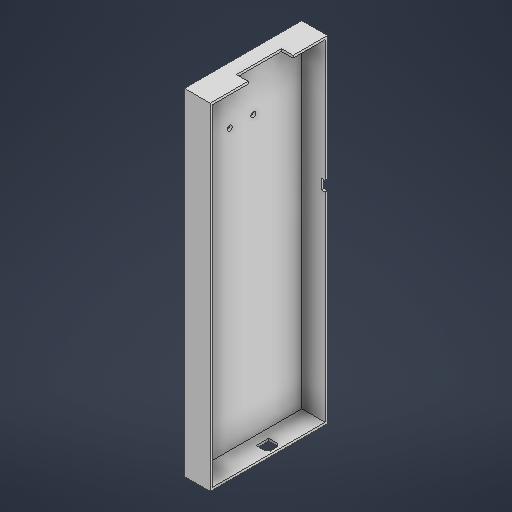
# Autodesk Inventor part: cDAQ_Bottom_Box3
Saved by Autodesk Inventor 2027 (Build 310192000, 192)
## iProperties
Created: 2026-05-08
Part Number: cDAQ_Bottom_Box3
Material: Generic
Document SubType Name: Modeling
Designer: giese
Density: 1 g/cm^3
Appearance: Default
Author: giese
Autodesk Inventor part; units mm, degrees
ref_plane "YZ Plane" through (0, 0, 0) normal (1, 0, 0) x (0, 1, 0)
ref_plane "XZ Plane" through (0, 0, 0) normal (0, 1, 0) x (-1, 0, 0)
ref_plane "XY Plane" through (0, 0, 0) normal (0, 0, 1) x (1, 0, 0)
sketch "Sketch1" plane through (0, 0, 0) normal (1, 0, 0) x (0, 1, 0)
  line L0 (37.5698, 44.2767) -> (-228.1396, 44.2767)
  line L1 (-228.1396, 44.2767) -> (-228.1396, -48.4333)
  line L2 (-228.1396, -48.4333) -> (37.5698, -48.4333)
  line L3 (37.5698, -48.4333) -> (37.5698, 44.2767)
  point P0 (0, 0)
  dimension "d0" = 92.71
  dimension "d1" = 265.7094
  constraints: 8 end point, 2 parallel, 1 horizontal, 1 perpendicular
  measures "d0" distance of L2.end L0.start
  measures "d1" distance of L1.end L2.end
extrude "Extrusion1" add sketch "Sketch1" along normal blind 20.32
sketch "Sketch2" plane through (20.32, 0, 0) normal (1, 0, 0) x (0, 0, -1)
  line L0 (46.5283, 35.6648) -> (-42.3717, 35.6648)
  line L1 (-42.3717, 35.6648) -> (-42.3717, -226.2346)
  line L2 (-42.3717, -226.2346) -> (46.5283, -226.2346)
  line L3 (46.5283, -226.2346) -> (46.5283, 35.6648)
  line L4 (48.4333, 37.5698) -> (-44.2767, 37.5698) projected
  line L5 (-44.2767, 37.5698) -> (-44.2767, -228.1396) projected
  point P0 (0, 0)
  dimension "d4" = 261.8994
  dimension "d5" = 88.9
  dimension "d8" = 1.905
  dimension "d21" = 1.905
  constraints: 8 end point, 2 parallel, 1 horizontal, 1 perpendicular
  measures "d4" distance of L2.end L0.start
  measures "d5" distance of L0.start L0.end
  measures "d8" distance between parallel lines of L0 L4
  measures "d21" distance between parallel lines of L5 L1
extrude "Extrusion2" cut sketch "Sketch2" against normal blind 18.415
sketch "Sketch3" plane through (0, 0, 0) normal (-1, 0, 0) x (0, 0, 1)
  circle A0 centre (-8.1895, -5.661) radius 2
  circle A1 centre (10.3093, -5.661) radius 2
  circle A2 centre (28.8081, -5.661) radius 2
  line L0 (-48.4333, -228.1396) -> (-48.4333, 37.5698) projected
  line L1 (-48.4333, 37.5698) -> (44.2767, 37.5698) projected
  line L2 (44.2767, 37.5698) -> (44.2767, -228.1396) projected
  line L3 (42.3717, 35.6648) -> (-46.5283, 35.6648) projected
  point P0 (0, 0)
  point P1 (-0.896, -23.7433)
  point P2 (-45.1848, 27.0137)
  dimension "d9" = 18.4988
  dimension "d10" = 4
  dimension "d11" = 4
  dimension "d12" = 18.4988
  dimension "d13" = 36.9976
  dimension "d18" = 15.4686
  dimension "d22" = 4
  dimension "d50" = 41.3258
  constraints: 3 centre point
  measures "d9" distance of A0.centre A1.centre
  measures "d10" diameter of A1
  measures "d11" diameter of A2
  measures "d12" distance of A1.centre A2.centre
  measures "d13" distance of A0.centre A2.centre
  measures "d18" distance from line of L2 A2.centre
  measures "d22" diameter of A0
  measures "d50" distance from line of L3 A2.centre
extrude "Extrusion3" cut sketch "Sketch3" against normal blind 3.81
sketch "Sketch5" plane through (0, -228.1396, -48.4333) normal (0, 0, -1) x (-1, 0, 0)
  line L0 (-20.32, 159.4866) -> (-17.4625, 159.4866)
  line L1 (-17.4625, 159.4866) -> (-17.4625, 167.4866)
  line L2 (-17.4625, 167.4866) -> (-20.32, 167.4866)
  line L3 (-20.32, 167.4866) -> (-20.32, 159.4866)
  line L4 (0, 265.7094) -> (-20.32, 265.7094) projected
  line L5 (0, 0) -> (0, 265.7094) projected
  point P0 (0, 228.1396)
  point P1 (-18.8913, 167.4866)
  point P2 (-18.8913, 159.4866)
  dimension "d28" = 2.8575
  dimension "d30" = 8
  dimension "d31" = 17.4625
  dimension "d34" = 106.2228
  constraints: 8 end point, 2 midpoint, 2 parallel, 1 horizontal, 1 perpendicular
  measures "d28" distance between parallel lines of L1 L3
  measures "d30" distance of point (-18.891, 167.487) point (-18.891, 159.487)
  measures "d31" distance between parallel lines of L5 L1
  measures "d34" distance between parallel lines of L4 L0
extrude "Extrusion4" cut sketch "Sketch5" against normal blind 24.13
sketch "Sketch6" plane through (0, -228.1396, -48.4333) normal (0, -1, 0) x (1, 0, 0)
  line L0 (16, 45.1284) -> (9, 45.1284)
  line L1 (9, 45.1284) -> (9, 35.1284)
  line L2 (9, 35.1284) -> (16, 35.1284)
  line L3 (0, 92.71) -> (0, 0) projected
  line L4 (18.24, 43.1283) -> (18.24, 37.1284)
  line L5 (16, 45.1284) -> (18.24, 43.1283)
  line L6 (18.24, 37.1284) -> (16, 35.1284)
  line L7 (0, 0) -> (20.32, 0) projected
  point P0 (0, 48.4333)
  point P1 (12.5, 45.1284)
  point P2 (12.5, 35.1284)
  dimension "d35" = 10
  dimension "d39" = 6
  dimension "d48" = 45.1284
  dimension "d49" = 18.24
  constraints: 12 end point, 2 midpoint, 1 horizontal, 1 parallel, 1 perpendicular, 1 vertical
  measures "d35" distance of point (12.5, 45.128) point (12.5, 35.128)
  measures "d39" distance of L4.start L4.end
  measures "d48" distance between parallel lines of L7 L0
  measures "d49" distance between parallel lines of L3 L4
extrude "Extrusion5" cut sketch "Sketch6" against normal blind 3.81
sketch "Sketch7" plane through (0, 37.5698, 44.2767) normal (0, 1, 0) x (1, 0, 0)
  line L0 (26.1366, 65.4812) -> (11.1252, 65.4812)
  line L1 (11.1252, 65.4812) -> (11.1252, 29.9212)
  line L2 (11.1252, 29.9212) -> (26.1366, 29.9212)
  line L3 (26.1366, 29.9212) -> (26.1366, 65.4812)
  line L4 (0, 0) -> (20.32, 0) projected
  line L5 (0, 92.71) -> (0, 0) projected
  line L6 (20.32, 92.71) -> (20.32, 0) projected
  point P0 (0, 44.2767)
  dimension "d51" = 35.56
  dimension "d52" = 29.9212
  dimension "d55" = 11.1252
  dimension "d56" = 15.0114
  dimension "d57" = 5.8166
  constraints: 8 end point, 2 parallel, 1 horizontal, 1 perpendicular
  measures "d51" distance of L2.end L0.start
  measures "d52" distance between parallel lines of L4 L2
  measures "d55" distance between parallel lines of L5 L1
  measures "d56" distance between parallel lines of L3 L1
  measures "d57" distance between parallel lines of L6 L3
extrude "Extrusion6" cut sketch "Sketch7" against normal blind 3.81
body "Solid1"
